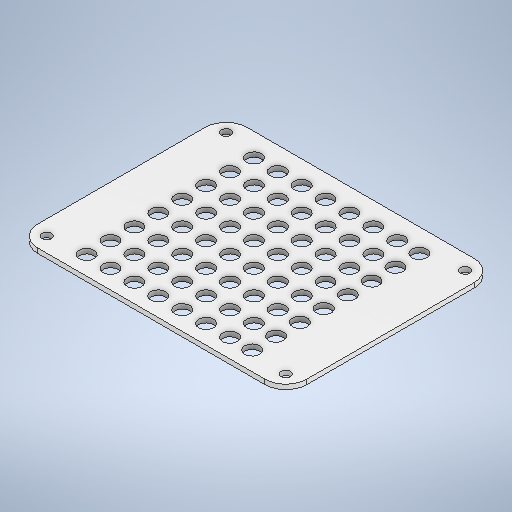
# Autodesk Inventor part: placa leds
Saved by Autodesk Inventor 2025 (Build 290162000, 162)
## iProperties
Created: 2024-04-28
Part Number: placa leds
Material: PPS Plastic
Document SubType Name: Modeling
Designer: kaike
Density: 1.637 g/cm^3
Appearance: Smooth - White
Mass: 13.0141 g
Surface Area: 121.035 cm^2
Volume: 7.95 cm^3
Author: kaike
Autodesk Inventor part; units mm, degrees
ref_plane "YZ Plane" through (0, 0, 0) normal (1, 0, 0) x (0, 1, 0)
ref_plane "XZ Plane" through (0, 0, 0) normal (0, 1, 0) x (-1, 0, 0)
ref_plane "XY Plane" through (0, 0, 0) normal (0, 0, 1) x (1, 0, 0)
sketch "Sketch1" plane through (0, 0, 0) normal (0, 1, 0) x (-1, 0, 0)
  line L0 (90, 0) -> (90, -70)
  line L1 (90, -70) -> (0, -70)
  line L2 (0, -70) -> (0, 0)
  line L3 (90, 0) -> (0, 0)
  circle A0 centre (85, -5) radius 1.6095
  circle A1 centre (85, -65) radius 1.6095
  circle A2 centre (72.9852, -6.2872) radius 2.5
  circle A3 centre (72.9852, -14.2872) radius 2.5
  circle A4 centre (72.9852, -22.2872) radius 2.5
  circle A5 centre (72.9852, -30.2872) radius 2.5
  circle A6 centre (72.9852, -38.2872) radius 2.5
  circle A7 centre (72.9852, -46.2872) radius 2.5
  circle A8 centre (72.9852, -54.2872) radius 2.5
  circle A9 centre (72.9852, -62.2872) radius 2.5
  circle A10 centre (64.9852, -6.2872) radius 2.5
  circle A11 centre (64.9852, -14.2872) radius 2.5
  circle A12 centre (64.9852, -22.2872) radius 2.5
  circle A13 centre (64.9852, -30.2872) radius 2.5
  circle A14 centre (64.9852, -38.2872) radius 2.5
  circle A15 centre (64.9852, -46.2872) radius 2.5
  circle A16 centre (64.9852, -54.2872) radius 2.5
  circle A17 centre (64.9852, -62.2872) radius 2.5
  circle A18 centre (56.9852, -6.2872) radius 2.5
  circle A19 centre (56.9852, -14.2872) radius 2.5
  circle A20 centre (56.9852, -22.2872) radius 2.5
  circle A21 centre (56.9852, -30.2872) radius 2.5
  circle A22 centre (56.9852, -38.2872) radius 2.5
  circle A23 centre (56.9852, -46.2872) radius 2.5
  circle A24 centre (56.9852, -54.2872) radius 2.5
  circle A25 centre (56.9852, -62.2872) radius 2.5
  circle A26 centre (48.9852, -6.2872) radius 2.5
  circle A27 centre (48.9852, -14.2872) radius 2.5
  circle A28 centre (48.9852, -22.2872) radius 2.5
  circle A29 centre (48.9852, -30.2872) radius 2.5
  circle A30 centre (48.9852, -38.2872) radius 2.5
  circle A31 centre (48.9852, -46.2872) radius 2.5
  circle A32 centre (48.9852, -54.2872) radius 2.5
  circle A33 centre (48.9852, -62.2872) radius 2.5
  circle A34 centre (40.9852, -6.2872) radius 2.5
  circle A35 centre (40.9852, -14.2872) radius 2.5
  circle A36 centre (40.9852, -22.2872) radius 2.5
  circle A37 centre (40.9852, -30.2872) radius 2.5
  circle A38 centre (40.9852, -38.2872) radius 2.5
  circle A39 centre (40.9852, -46.2872) radius 2.5
  circle A40 centre (40.9852, -54.2872) radius 2.5
  circle A41 centre (40.9852, -62.2872) radius 2.5
  circle A42 centre (32.9852, -6.2872) radius 2.5
  circle A43 centre (32.9852, -14.2872) radius 2.5
  circle A44 centre (32.9852, -22.2872) radius 2.5
  circle A45 centre (32.9852, -30.2872) radius 2.5
  circle A46 centre (32.9852, -38.2872) radius 2.5
  circle A47 centre (32.9852, -46.2872) radius 2.5
  circle A48 centre (32.9852, -54.2872) radius 2.5
  circle A49 centre (32.9852, -62.2872) radius 2.5
  circle A50 centre (24.9852, -6.2872) radius 2.5
  circle A51 centre (24.9852, -14.2872) radius 2.5
  circle A52 centre (24.9852, -22.2872) radius 2.5
  circle A53 centre (24.9852, -30.2872) radius 2.5
  circle A54 centre (24.9852, -38.2872) radius 2.5
  circle A55 centre (24.9852, -46.2872) radius 2.5
  circle A56 centre (24.9852, -54.2872) radius 2.5
  circle A57 centre (24.9852, -62.2872) radius 2.5
  circle A58 centre (17.5855, -6.2872) radius 2.5
  circle A59 centre (17.5855, -14.2872) radius 2.5
  circle A60 centre (17.5855, -22.2872) radius 2.5
  circle A61 centre (17.5855, -30.2872) radius 2.5
  circle A62 centre (17.5855, -38.2872) radius 2.5
  circle A63 centre (17.5855, -46.2872) radius 2.5
  circle A64 centre (17.5855, -54.2872) radius 2.5
  circle A65 centre (17.5855, -62.2872) radius 2.5
  circle A66 centre (5, -5) radius 1.6095
  circle A67 centre (5, -65) radius 1.6095
  dimension "d27" = 60
  dimension "d28" = 5
  dimension "d29" = 5
  dimension "d30" = 55.3996
  dimension "d33" = 56
  dimension "d34" = 5
  dimension "d35" = 8
  dimension "d36" = 3
  dimension "d37" = 3
  dimension "d38" = 90
  dimension "d39" = 3.219
  constraints: 68 centre point, 8 end point, 2 perpendicular, 1 horizontal, 1 vertical
  measures "d27" distance of A1.centre A0.centre
  measures "d28" distance from line of L0 A1.centre
  measures "d29" distance from line of L1 A1.centre
  measures "d30" distance of A58.centre A2.centre
  measures "d33" distance of A58.centre A65.centre
  measures "d34" diameter of A9
  measures "d35" distance of A3.centre A2.centre
  measures "d38" distance of L0.end L1.end
  measures "d39" diameter of A0
extrude "Extrusion1" add sketch "Sketch1" along normal blind 1.6
fillet "Fillet1" radius 7 4 edges at (0, 0.8, 0) (-90, 0.8, 0) (0, 0.8, -70) (-90, 0.8, -70)
body "Solid1"
